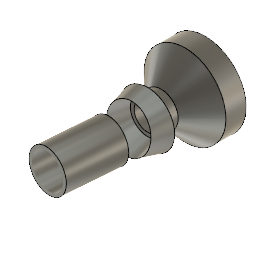
cpeg398 final stuff (Autodesk Fusion 360 design; units mm, degrees)
Autodesk Fusion 360 part; units mm, degrees
sketch "Sketch1" plane through (0, 0, 0) normal (0, 0, 1) x (1, 0, 0)
sketch "Sketch1 (2)" plane through (0, 0, 0) normal (0, 1, 0) x (1, 0, 0) in component "Circle"
  circle A0 centre (0, -2.4593) radius 25.1207
extrude "Extrude1" add sketch "Sketch1 (2)" along normal blind 35 draft 45 makes body 1 in component "Circle"
sketch "Sketch2" plane through (0, 0, 0) normal (0, -1, 0) x (1, 0, 0) in component "Circle"
  circle A0 centre (0, 2.4593) radius 25.1207
  circle A1 centre (0, 2.4593) radius 19.5517
extrude "Extrude2" cut sketch "Sketch2" against normal blind 45 contours A1 bodies 1 in component "Circle"
extrude "Extrude3" add 1 faces at (23.098, 0, 4.6787) along direction (0, -1, 0) blind 20 on bodies 1 bodies 1 in component "Circle"
sketch "Sketch1 (3)" plane through (0, 0, 0) normal (1, 0, 0) x (0, 1, 0) in component "Connector"
  circle A0 centre (-75, 0) radius 25
  circle A1 centre (-75, 0) radius 30
extrude "Extrude1'" add sketch "Sketch1 (3)" along normal blind 85 separate body makes body 2 in component "Connector"
move_body "MoveFace1" bodies 2 to x (-0.080521, -0.996752, -0.001074) y (0.907488, -0.073756, 0.413552) z (-0.412289, 0.032325, 0.91048) at (68.0616, -80.5317, 31.0164) on bodies 2 in component "Connector"
sketch "Sketch2 (2)" plane through (0, -20, 0) normal (0, -1, 0) x (1, 0, 0)
  circle A0 centre (0, 2.4593) radius 19.5517
  circle A1 centre (0, 2.4593) radius 25.1207
  circle A2 centre (0, 0) radius 40
  circle A3 centre (0, 0) radius 21.9892
extrude "Extrude1''" add sketch "Sketch2 (2)" along normal blind 40 draft -15 separate body contours A2 makes body 3
sketch "Sketch3" plane through (0, 35, 0) normal (0, 1, 0) x (-1, 0, 0)
  circle A0 centre (0, 2.4593) radius 19.5517
  circle A1 centre (0, 2.4593) radius 60.1207
  circle A2 centre (0, 2.5) radius 55.0568
extrude "Extrude4" add sketch "Sketch3" along normal blind 30 contours A1 bodies 1 in component "Circle"
component "Circle" placed x (1, 0, 0) y (0, 1, 0) z (0, 0, 1) at (0, 0, 0)
component "Connector" placed x (1, 0, 0) y (0, 1, 0) z (0, 0, 1) at (0, 0, 0)
